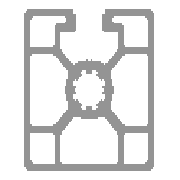
# Autodesk Inventor part: 3 842 992 401-25mm
Saved by Autodesk Inventor 2011 SP1 (Build 150282100, 282)
## iProperties
Category: End -/-
Created: 2011-02-21
Part Number: 3 842 992 401-25mm
Document SubType Name: Modeling
Designer: SRW
Density: 2.71 g/cm^3
Categories: <MemberInstance><Categories><Category DisplayName="Structural Shapes" InternalName="089c4875-fa83-4c05-b084-43b9cc11f5ed" Mnemonic="GRDR"><CategoryParameter DisplayName="Custom Base Point" InternalName="4f1d1b73-316d-484b-a3df-9cbabb16eb77" Mnemonic="shpBasePoint"/><CategoryParameter DisplayName="FG Authored" InternalName="9c666724-f362-4ea7-ac62-f6a007de5c69" Mnemonic="shpFGAuto"/><CategoryParameter DisplayName="Legacy Member ID" InternalName="340afe4f-75d7-48d3-ab7d-943f3c3da468" Mnemonic="LegacyMemberID"/><CategoryParameter DisplayName="Base Length" InternalName="42e34263-8f20-4d0e-ad48-bf1385b87c24" Mnemonic="shplen"/><CategoryParameter DisplayName="Distance of the Center of Gravity X-X" InternalName="26c9bdb8-9c79-4b4f-a92e-8e197583c9c4" Mnemonic="grcendistX"/><CategoryParameter DisplayName="Distance of the Center of Gravity Y-Y" InternalName="bcc4fb17-7af4-436a-8f8c-d0aa3b0248c5" Mnemonic="grcendistY"/><CategoryParameter DisplayName="Torsional Rigidity Modulus" InternalName="26c1ec35-5026-4c63-ad0a-751cf684a536" Mnemonic="torrigmod"/><CategoryParameter DisplayName="Torsional Section Modulus" InternalName="7c55a8dc-8844-49f9-a867-cc677b30ec9a" Mnemonic="torsecmod"/><CategoryParameter DisplayName="Coefficient of Shear Displacement" InternalName="de4c90c6-aaa8-468f-a335-6737b311b5d3" Mnemonic="shdispc"/><CategoryParameter DisplayName="Section Area" InternalName="1ff91680-64b0-4202-b9a3-7fd3f94bba3b" Mnemonic="secarea"/><CategoryParameter DisplayName="Moment of Inertia (x)" InternalName="4cd780bc-73d7-43ac-917a-579e5cbd684d" Mnemonic="inermomx"/><CategoryParameter DisplayName="Moment of Inertia (y)" InternalName="4b9f58ea-bced-460e-81ea-3d29ca5a49e3" Mnemonic="inermomy"/><CategoryParameter DisplayName="Section Module (x)" InternalName="72cfad18-cf51-4ed4-aaa7-c6b224f8419f" Mnemonic="secmodx"/><CategoryParameter DisplayName="Section Module (y)" InternalName="59eaa5e9-d227-48dc-b6c1-6920f96e0f95" Mnemonic="secmody"/><CategoryParameter DisplayName="Radius of Gyration (x)" InternalName="25778675-03e9-40c1-b6a8-4a9ed693320d" Mnemonic="gyrradx"/><CategoryParameter DisplayName="Radius of Gyration (y)" InternalName="bfa18ebe-1636-4dbe-8d42-b263e0b73184" Mnemonic="gyrrady"/><CategoryParameter DisplayName="Shape Thickness" InternalName="d109cf76-8eb4-42fc-9800-4409734adc67" Mnemonic="shpthick"/><CategoryParameter DisplayName="Second Shape Thickness" InternalName="9251a8e1-85fd-4e47-af99-afdb762317d9" Mnemonic="shpthick2"/><CategoryParameter DisplayName="Shape Width" InternalName="7c717d54-a18f-4666-b4d4-573cce22c62c" Mnemonic="shpwdth"/><CategoryParameter DisplayName="Shape Height" InternalName="50274e7d-5ac0-4796-92cb-c59e54983c67" Mnemonic="shpheig"/><CategoryParameter DisplayName="Mass per Length Unit" InternalName="0bb95a10-148f-4027-a459-38d7b056702a" Mnemonic="shpmass"/><CategoryParameter DisplayName="Section Designation" InternalName="5a64d034-428d-49c8-ba32-7619764de20f" Mnemonic="shpdes"/><Category DisplayName="Other" InternalName="f02205ff-2390-476f-921c-0b3185f88e84" Mnemonic="OTHSHP"><CategoryParameter DisplayName="Moment of Inertia (x)" InternalName="ec6737bc-264f-43ed-b0bd-f6d410c2718d" Mnemonic="inermomx"/><CategoryParameter DisplayName="Moment of Inertia (y)" InternalName="044c654e-f649-48ac-84cc-650a29ae31ca" Mnemonic="inermomy"/><CategoryParameter DisplayName="Section Module (x)" InternalName="cac70804-9d39-43bb-be17-56ea1f39a6c2" Mnemonic="secmodx"/><CategoryParameter DisplayName="Section Module (y)" InternalName="88b8bff9-a616-4028-93d5-ed4f79680d13" Mnemonic="secmody"/><CategoryParameter DisplayName="Section Area" InternalName="c46ecdf8-b6eb-4db9-8b25-30258930c1e3" Mnemonic="secarea"/><CategoryParameter DisplayName="Radius of Gyration (x)" InternalName="ee72c61e-565e-4fd6-b448-66e1e1abcb7e" Mnemonic="gyrradx"/><CategoryParameter DisplayName="Radius of Gyration (y)" InternalName="743e1dfe-1bba-408b-b985-cf752b207386" Mnemonic="gyrrady"/><CategoryParameter DisplayName="Shape Thickness" InternalName="12b1a788-9233-48fd-a933-2df8ff42b15f" Mnemonic="shpthick"/><CategoryParameter DisplayName="Mass per Length Unit" InternalName="2fd289d6-9394-4d2d-97e6-6659d7d4551d" Mnemonic="shpmass"/></Category></Category></Categories><FamilyTemplate Id="45x45 1S"><FamilyTemplateParameters><FamilyTemplateParameter ObjectType="kUserParameterObject" ValueType="xs:double" Id="9" ObjectReferenceKey="G_L"/><FamilyTemplateParameter ObjectType="kUserParameterObject" ValueType="xs:double" Id="10" ObjectReferenceKey="G_OFFSET_END"/><FamilyTemplateParameter ObjectType="kUserParameterObject" ValueType="xs:double" Id="11" ObjectReferenceKey="G_OFFSET_START"/><FamilyTemplateParameter ObjectType="kUserParameterObject" ValueType="xs:double" Id="12" ObjectReferenceKey="Length"/><FamilyTemplateParameter ObjectType="kPartFeatureObject" ValueType="xs:boolean" Id="1" ObjectReferenceKey="10020000100000001d0d0000000000008000000000000000" SubObjectId="Suppressed"/><FamilyTemplateParameter ObjectType="kPartFeatureObject" ValueType="xs:boolean" Id="2" ObjectReferenceKey="1002000010000000c00e0000000000008000000000000000" SubObjectId="Suppressed"/><FamilyTemplateParameter ObjectType="kPartFeatureObject" ValueType="xs:boolean" Id="3" ObjectReferenceKey="1002000010000000930f0000000000008000000000000000" SubObjectId="Suppressed"/><FamilyTemplateParameter ObjectType="kPartFeatureObject" ValueType="xs:boolean" Id="4" ObjectReferenceKey="1002000010000000180b0000000000008000000000000000" SubObjectId="Suppressed"/><FamilyTemplateParameter ObjectType="kPartFeatureObject" ValueType="xs:boolean" Id="6" ObjectReferenceKey="1002000010000000330c0000000000008000000000000000" SubObjectId="Suppressed"/><FamilyTemplateParameter ObjectType="kPartFeatureObject" ValueType="xs:boolean" Id="7" ObjectReferenceKey="1002000010000000f40d0000000000008000000000000000" SubObjectId="Suppressed"/><FamilyTemplateParameter ObjectType="kPartFeatureObject" ValueType="xs:boolean" Id="8" ObjectReferenceKey="10020000100000008b160000000000008000000000000000" SubObjectId="Suppressed"/><FamilyTemplateParameter ObjectType="kPartFeatureObject" ValueType="xs:boolean" Id="13" ObjectReferenceKey="1002000010000000590a0000000000008000000000000000" SubObjectId="Suppressed"/><FamilyTemplateParameter ObjectType="kPropertyObject" ValueType="xs:string" Id="16" ObjectReferenceKey="{D5CDD502-2E9C-101B-9397-08002B2CF9AE}" SubObjectId="2"/><FamilyTemplateParameter ObjectType="kPropertyObject" ValueType="xs:string" Id="17" ObjectReferenceKey="{32853F0F-3444-11d1-9E93-0060B03C1CA6}" SubObjectId="52"/><FamilyTemplateParameter ObjectType="kPartComponentDefinitionObject" ValueType="xs:string" Id="18" SubObjectId="Material"/><FamilyTemplateParameter ObjectType="kPropertyObject" ValueType="xs:string" Id="19" ObjectReferenceKey="{32853F0F-3444-11d1-9E93-0060B03C1CA6}" SubObjectId="5"/><FamilyTemplateParameter ObjectType="kPropertyObject" ValueType="xs:string" Id="20" ObjectReferenceKey="{32853F0F-3444-11D1-9E93-0060B03C1CA6}" SubObjectId="55"/><FamilyTemplateParameter ObjectType="kiPartTableColumnObject" ValueType="xs:string" Id="29" ObjectReferenceKey="FILENAME"/><FamilyTemplateParameter ObjectType="kiPartTableColumnObject" ValueType="xs:string" Id="30" ObjectReferenceKey="MEMBER_REVISION"/></FamilyTemplateParameters></FamilyTemplate><CategoryParameterMap><ParamToTemplateMap><ParamToTemplate CategoryParameter="//CategoryParameter[@InternalName='2675968c-4ce5-49e0-a4f5-552d29089031']" TemplateParameter="17"/><ParamToTemplate CategoryParameter="//CategoryParameter[@InternalName='8b46a4cc-9585-4fed-90c3-899f57e09a73']" TemplateParameter="29"/><ParamToTemplate CategoryParameter="//CategoryParameter[@InternalName='42e34263-8f20-4d0e-ad48-bf1385b87c24']" TemplateParameter="12"/><ParamToTemplate CategoryParameter="//CategoryParameter[@InternalName='818a152a-d3c3-49ca-80ee-df7d91421b8e']" TemplateParameter="18"/><ParamToTemplate CategoryParameter="//CategoryParameter[@InternalName='a65d44b9-392f-4f4f-857b-e4b3d54996fe']" TemplateParameter="30"/><ParamToTemplate CategoryParameter="//CategoryParameter[@InternalName='016b6077-bfbe-49bd-92c9-d8d59c39c941']" TemplateParameter="19"/><ParamToTemplate CategoryParameter="//CategoryParameter[@InternalName='9c666724-f362-4ea7-ac62-f6a007de5c69']" ConstantValue="1"/></ParamToTemplateMap></CategoryParameterMap></MemberInstance>
Stock Number: 3 842 992 401
Description: PROFILE 45x45 1S, -/-
Material: Aluminum-6061
Mass: 39.9838 g
Surface Area: 162.834 cm^2
Volume: 14.7542 cm^3
G_L: 25.000 mm
Author: SRW
Autodesk Inventor part; units mm, degrees
ref_plane "YZ Plane" through (0, 0, 0) normal (1, 0, 0) x (0, 1, 0)
ref_plane "XZ Plane" through (0, 0, 0) normal (0, 1, 0) x (-1, 0, 0)
sketch "45x45 1S" plane through (0, 0, 0) normal (0, 0, 1) x (1, 0, 0)
  line L0 (49.3347, 47.491) -> (36.1347, 47.491)
  arc A0 (36.1347, 47.491) -> (35.6347, 46.991) centre (36.1347, 46.991) ccw
  line L1 (35.6347, 46.991) -> (35.6347, 46.291)
  line L2 (35.3347, 45.991) -> (35.1347, 45.991)
  arc A1 (35.3347, 45.991) -> (35.6347, 46.291) centre (35.3347, 46.291) ccw
  line L3 (48.2375, 45.841) -> (38.8875, 45.841)
  arc A2 (35.1347, 45.991) -> (34.8347, 45.691) centre (35.1347, 45.691) ccw
  arc A3 (52.3347, 44.491) -> (49.3347, 47.491) centre (49.3347, 44.491) ccw
  arc A4 (50.7375, 43.341) -> (48.2375, 45.841) centre (48.2375, 43.341) ccw
  arc A5 (38.8875, 45.841) -> (38.8875, 43.141) centre (38.8875, 44.491) ccw
  line L4 (38.8875, 43.141) -> (40.5875, 43.141)
  line L5 (34.8347, 45.691) -> (34.8347, 41.691)
  arc A6 (34.8347, 41.691) -> (35.0347, 41.491) centre (35.0347, 41.691) ccw
  line L6 (35.0347, 41.491) -> (39.6847, 41.491)
  arc A7 (39.8847, 41.291) -> (39.6847, 41.491) centre (39.6847, 41.291) ccw
  line L7 (41.5875, 42.141) -> (41.5875, 37.691)
  line L8 (50.7375, 37.691) -> (50.7375, 43.341)
  line L9 (39.8847, 41.291) -> (39.8847, 36.8066)
  line L10 (42.5875, 36.691) -> (49.7375, 36.691)
  arc A8 (49.7375, 36.691) -> (50.7375, 37.691) centre (49.7375, 37.691) ccw
  arc A9 (41.5875, 37.691) -> (42.5875, 36.691) centre (42.5875, 37.691) ccw
  arc A10 (41.5875, 42.141) -> (40.5875, 43.141) centre (40.5875, 42.141) ccw
  line L11 (50.7375, 15.941) -> (50.7375, 34.041)
  arc A11 (50.7375, 34.041) -> (49.7375, 35.041) centre (49.7375, 34.041) ccw
  line L12 (49.7375, 35.041) -> (42.4984, 35.041)
  arc A12 (42.4984, 35.041) -> (41.0842, 34.4553) centre (42.4984, 33.041) ccw
  arc A13 (39.2989, 35.3924) -> (39.8847, 36.8066) centre (37.8847, 36.8066) ccw
  line L13 (41.0842, 34.4553) -> (37.447, 30.8181)
  arc A14 (37.447, 30.8181) -> (37.0665, 28.5213) centre (38.8612, 29.4039) ccw
  line L14 (39.2989, 35.3924) -> (36.4578, 32.5512)
  arc A15 (37.0665, 21.4608) -> (37.0665, 28.5213) centre (29.8875, 24.991) ccw
  line L15 (52.3347, 5.491) -> (52.3347, 44.491)
  arc A16 (30.7383, 32.991) -> (30.614, 32.9554) centre (30.7353, 32.767) ccw
  arc A17 (34.161, 32.1707) -> (30.7383, 32.991) centre (30.6307, 24.9918) ccw
  arc A18 (34.161, 32.1707) -> (36.4578, 32.5512) centre (35.0436, 33.9654) ccw
  arc A19 (35.7235, 23.3997) -> (35.3276, 24.0225) centre (35.2408, 23.5301) ccw
  arc A20 (35.3276, 25.9596) -> (35.7235, 26.5824) centre (35.2408, 26.452) ccw
  arc A21 (35.124, 21.9524) -> (35.7235, 23.3997) centre (29.8347, 24.991) ccw
  arc A22 (35.7235, 26.5824) -> (35.124, 28.0297) centre (29.8347, 24.991) ccw
  line L16 (34.81, 25.8683) -> (35.3276, 25.9596)
  line L17 (35.3276, 24.0225) -> (34.81, 24.1138)
  arc A23 (34.81, 24.1138) -> (34.81, 25.8683) centre (29.8875, 24.991) ccw
  arc A24 (34.4036, 21.7918) -> (35.124, 21.9524) centre (34.6904, 22.2014) ccw
  line L18 (34.4036, 28.1902) -> (33.9658, 27.8837)
  line L19 (33.9658, 22.0984) -> (34.4036, 21.7918)
  arc A25 (32.8734, 19.7018) -> (33.0339, 20.4221) centre (32.6243, 20.1353) ccw
  line L20 (33.0339, 20.4221) -> (32.7199, 20.8706)
  arc A26 (32.7199, 20.8706) -> (33.9658, 22.0984) centre (29.8875, 24.991) ccw
  arc A27 (31.4261, 19.1023) -> (32.8734, 19.7018) centre (29.8347, 24.991) ccw
  arc A28 (29.8347, 17.0144) -> (33.3735, 17.8163) centre (29.8875, 24.991) ccw
  arc A29 (30.8033, 19.4982) -> (31.4261, 19.1023) centre (31.2957, 19.585) ccw
  line L21 (30.703, 20.067) -> (30.8033, 19.4982)
  arc A30 (33.0867, 29.56) -> (32.8734, 30.2803) centre (32.6637, 29.8264) ccw
  arc A31 (33.9658, 27.8837) -> (32.7554, 29.0868) centre (29.8875, 24.991) ccw
  line L22 (32.7554, 29.0868) -> (33.0867, 29.56)
  arc A32 (32.8734, 30.2803) -> (31.4261, 30.8798) centre (29.8347, 24.991) ccw
  arc A33 (31.4261, 30.8798) -> (30.8033, 30.4839) centre (31.2957, 30.3971) ccw
  line L23 (30.8033, 30.4839) -> (30.7045, 29.9238)
  arc A34 (35.124, 28.0297) -> (34.4036, 28.1902) centre (34.6904, 27.7807) ccw
  arc A35 (49.3347, 2.491) -> (52.3347, 5.491) centre (49.3347, 5.491) ccw
  arc A36 (39.8847, 12.3802) -> (39.2989, 13.7944) centre (37.8847, 12.3802) ccw
  arc A37 (49.7375, 14.941) -> (50.7375, 15.941) centre (49.7375, 15.941) ccw
  line L24 (42.4984, 14.941) -> (49.7375, 14.941)
  arc A38 (41.0841, 15.5268) -> (42.4984, 14.941) centre (42.4984, 16.941) ccw
  line L25 (39.8847, 5.141) -> (39.8847, 12.3802)
  arc A39 (42.5875, 13.291) -> (41.5875, 12.291) centre (42.5875, 12.291) ccw
  line L26 (49.7375, 13.291) -> (42.5875, 13.291)
  arc A40 (50.7375, 12.291) -> (49.7375, 13.291) centre (49.7375, 12.291) ccw
  arc A41 (38.8847, 4.141) -> (39.8847, 5.141) centre (38.8847, 5.141) ccw
  line L27 (41.5875, 12.291) -> (41.5875, 5.141)
  arc A42 (41.5875, 5.141) -> (42.5875, 4.141) centre (42.5875, 5.141) ccw
  line L28 (50.7375, 6.641) -> (50.7375, 12.291)
  line L29 (42.5875, 4.141) -> (48.2375, 4.141)
  arc A43 (48.2375, 4.141) -> (50.7375, 6.641) centre (48.2375, 6.641) ccw
  arc A44 (23.2117, 32.5512) -> (25.5085, 32.1707) centre (24.6259, 33.9654) ccw
  arc A45 (28.9312, 32.991) -> (25.5085, 32.1707) centre (29.0387, 24.9918) ccw
  arc A46 (29.0555, 32.9554) -> (28.9312, 32.991) centre (28.9342, 32.767) ccw
  line L30 (29.7348, 32.5178) -> (29.0555, 32.9554)
  arc A47 (25.2658, 28.1902) -> (24.5455, 28.0297) centre (24.979, 27.7807) ccw
  arc A48 (26.796, 30.2803) -> (26.5827, 29.56) centre (27.0058, 29.8264) ccw
  line L31 (25.7036, 27.8837) -> (25.2658, 28.1902)
  arc A49 (29.7348, 32.5178) -> (29.8347, 32.491) centre (29.8348, 32.691) ccw
  arc A50 (29.8347, 32.491) -> (29.9347, 32.5178) centre (29.8347, 32.691) ccw
  line L32 (30.614, 32.9554) -> (29.9347, 32.5178)
  arc A51 (24.5455, 28.0297) -> (23.946, 26.5824) centre (29.8347, 24.991) ccw
  arc A52 (28.2433, 30.8798) -> (26.796, 30.2803) centre (29.8347, 24.991) ccw
  arc A53 (28.8662, 30.4839) -> (28.2433, 30.8798) centre (28.3738, 30.3971) ccw
  arc A54 (23.946, 26.5824) -> (24.3419, 25.9596) centre (24.4287, 26.452) ccw
  arc A55 (26.914, 29.0868) -> (25.7036, 27.8837) centre (29.7819, 24.991) ccw
  line L33 (28.965, 29.9238) -> (28.8662, 30.4839)
  line L34 (24.3419, 25.9596) -> (24.8595, 25.8683)
  arc A56 (29.8347, 29.9908) -> (28.965, 29.9238) centre (29.7819, 24.991) ccw
  arc A57 (30.7045, 29.9238) -> (29.8347, 29.9908) centre (29.8875, 24.991) ccw
  arc A58 (24.8595, 25.8683) -> (24.8595, 24.1138) centre (29.7819, 24.991) ccw
  line L35 (24.8595, 24.1138) -> (24.3419, 24.0225)
  arc A59 (24.3419, 24.0225) -> (23.946, 23.3997) centre (24.4287, 23.5301) ccw
  arc A60 (22.603, 28.5213) -> (22.603, 21.4608) centre (29.7819, 24.991) ccw
  arc A61 (23.946, 23.3997) -> (24.5455, 21.9524) centre (29.8347, 24.991) ccw
  arc A62 (24.5455, 21.9524) -> (25.2658, 21.7918) centre (24.979, 22.2014) ccw
  line L36 (25.2658, 21.7918) -> (25.7036, 22.0984)
  line L37 (26.5827, 29.56) -> (26.914, 29.0868)
  arc A63 (10.3347, 47.491) -> (7.3348, 44.491) centre (10.3347, 44.491) ccw
  line L38 (23.5348, 47.491) -> (10.3347, 47.491)
  arc A64 (24.0348, 46.991) -> (23.5348, 47.491) centre (23.5348, 46.991) ccw
  line L39 (24.0348, 46.291) -> (24.0348, 46.991)
  arc A65 (24.0348, 46.291) -> (24.3348, 45.991) centre (24.3348, 46.291) ccw
  line L40 (24.5348, 45.991) -> (24.3348, 45.991)
  arc A66 (24.8348, 45.691) -> (24.5348, 45.991) centre (24.5348, 45.691) ccw
  line L41 (24.8348, 41.691) -> (24.8348, 45.691)
  arc A67 (24.6348, 41.491) -> (24.8348, 41.691) centre (24.6348, 41.691) ccw
  line L42 (19.9848, 41.491) -> (24.6348, 41.491)
  arc A68 (19.9848, 41.491) -> (19.7848, 41.291) centre (19.9848, 41.291) ccw
  line L43 (19.7848, 36.8066) -> (19.7848, 41.291)
  arc A69 (19.7848, 36.8066) -> (20.3705, 35.3924) centre (21.7848, 36.8066) ccw
  arc A70 (17.0819, 36.691) -> (18.0819, 37.691) centre (17.0819, 37.691) ccw
  line L44 (18.0819, 37.691) -> (18.0819, 42.141)
  line L45 (9.9319, 36.691) -> (17.0819, 36.691)
  line L46 (19.0819, 43.141) -> (20.7819, 43.141)
  arc A71 (19.0819, 43.141) -> (18.0819, 42.141) centre (19.0819, 42.141) ccw
  arc A72 (8.9319, 37.691) -> (9.9319, 36.691) centre (9.9319, 37.691) ccw
  arc A73 (20.7819, 43.141) -> (20.7819, 45.841) centre (20.7819, 44.491) ccw
  line L47 (20.7819, 45.841) -> (11.4319, 45.841)
  arc A74 (11.4319, 45.841) -> (8.9319, 43.341) centre (11.4319, 43.341) ccw
  line L48 (8.9319, 43.341) -> (8.9319, 37.691)
  line L49 (10.3347, 2.491) -> (49.3347, 2.491)
  line L50 (37.447, 19.164) -> (41.0841, 15.5268)
  arc A75 (37.0665, 21.4608) -> (37.447, 19.164) centre (38.8612, 20.5782) ccw
  arc A76 (17.0819, 4.141) -> (18.0819, 5.141) centre (17.0819, 5.141) ccw
  arc A77 (18.0819, 12.291) -> (17.0819, 13.291) centre (17.0819, 12.291) ccw
  line L51 (18.0819, 5.141) -> (18.0819, 12.291)
  arc A78 (35.6618, 17.4316) -> (33.3735, 17.8163) centre (34.2476, 16.0174) ccw
  line L52 (39.2989, 13.7944) -> (35.6618, 17.4316)
  line L53 (20.7848, 4.141) -> (38.8847, 4.141)
  arc A79 (19.7848, 5.141) -> (20.7848, 4.141) centre (20.7848, 5.141) ccw
  line L54 (19.7848, 12.3802) -> (19.7848, 5.141)
  arc A80 (20.3705, 13.7944) -> (19.7848, 12.3802) centre (21.7848, 12.3802) ccw
  arc A81 (25.7036, 22.0984) -> (26.9496, 20.8706) centre (29.7819, 24.991) ccw
  arc A82 (28.9665, 20.067) -> (30.703, 20.067) centre (29.8347, 24.9911) ccw
  line L55 (26.9496, 20.8706) -> (26.6355, 20.4221)
  line L56 (28.8662, 19.4982) -> (28.9665, 20.067)
  arc A83 (26.796, 19.7018) -> (28.2433, 19.1023) centre (29.8347, 24.991) ccw
  arc A84 (28.2433, 19.1023) -> (28.8662, 19.4982) centre (28.3738, 19.585) ccw
  arc A85 (26.2959, 17.8163) -> (29.8347, 17.0144) centre (29.7819, 24.991) ccw
  arc A86 (22.2225, 19.164) -> (22.603, 21.4608) centre (20.8083, 20.5782) ccw
  arc A87 (26.2959, 17.8163) -> (24.0077, 17.4316) centre (25.4219, 16.0174) ccw
  line L57 (18.5853, 15.5268) -> (22.2225, 19.164)
  arc A88 (17.1711, 14.941) -> (18.5853, 15.5268) centre (17.1711, 16.941) ccw
  line L58 (24.0077, 17.4316) -> (20.3705, 13.7944)
  arc A89 (26.6355, 20.4221) -> (26.796, 19.7018) centre (27.0451, 20.1353) ccw
  arc A90 (7.3348, 5.491) -> (10.3347, 2.491) centre (10.3347, 5.491) ccw
  line L59 (7.3348, 44.491) -> (7.3348, 5.491)
  line L60 (23.2117, 32.5512) -> (20.3705, 35.3924)
  line L61 (11.4319, 4.141) -> (17.0819, 4.141)
  arc A91 (8.9319, 6.641) -> (11.4319, 4.141) centre (11.4319, 6.641) ccw
  line L62 (8.9319, 12.291) -> (8.9319, 6.641)
  arc A92 (9.9319, 13.291) -> (8.9319, 12.291) centre (9.9319, 12.291) ccw
  line L63 (17.0819, 13.291) -> (9.9319, 13.291)
  line L64 (9.9319, 14.941) -> (17.1711, 14.941)
  arc A93 (8.9319, 15.941) -> (9.9319, 14.941) centre (9.9319, 15.941) ccw
  line L65 (8.9319, 34.041) -> (8.9319, 15.941)
  line L66 (22.2225, 30.8181) -> (18.5853, 34.4553)
  arc A94 (18.5853, 34.4553) -> (17.1711, 35.041) centre (17.1711, 33.041) ccw
  line L67 (17.1711, 35.041) -> (9.9319, 35.041)
  arc A95 (9.9319, 35.041) -> (8.9319, 34.041) centre (9.9319, 34.041) ccw
  arc A96 (22.603, 28.5213) -> (22.2225, 30.8181) centre (20.8083, 29.4039) ccw
ref_plane "Start Plane" through (0, 0, 0) normal (0, 0, 1) x (1, 0, 0)
ref_plane "End Plane" through (0, 0, 25) normal (0, 0, 1) x (1, 0, 0)
sketch "Sketch1" plane through (0, 0, 0) normal (0, 0, 1) x (1, 0, 0)
  line L0 (19.5, 22.5) -> (6.3, 22.5)
  arc A0 (6.3, 22.5) -> (5.8, 22) centre (6.3, 22) ccw
  line L1 (5.8, 22) -> (5.8, 21.3)
  line L2 (5.5, 21) -> (5.3, 21)
  arc A1 (5.5, 21) -> (5.8, 21.3) centre (5.5, 21.3) ccw
  line L3 (18.4028, 20.85) -> (9.0528, 20.85)
  arc A2 (5.3, 21) -> (5, 20.7) centre (5.3, 20.7) ccw
  arc A3 (22.5, 19.5) -> (19.5, 22.5) centre (19.5, 19.5) ccw
  arc A4 (20.9028, 18.35) -> (18.4028, 20.85) centre (18.4028, 18.35) ccw
  arc A5 (9.0528, 20.85) -> (9.0528, 18.15) centre (9.0528, 19.5) ccw
  line L4 (9.0528, 18.15) -> (10.7528, 18.15)
  line L5 (5, 20.7) -> (5, 16.7)
  arc A6 (5, 16.7) -> (5.2, 16.5) centre (5.2, 16.7) ccw
  line L6 (5.2, 16.5) -> (9.85, 16.5)
  arc A7 (10.05, 16.3) -> (9.85, 16.5) centre (9.85, 16.3) ccw
  line L7 (11.7528, 17.15) -> (11.7528, 12.7)
  line L8 (20.9028, 12.7) -> (20.9028, 18.35)
  line L9 (10.05, 16.3) -> (10.05, 11.8156)
  line L10 (12.7528, 11.7) -> (19.9028, 11.7)
  arc A8 (19.9028, 11.7) -> (20.9028, 12.7) centre (19.9028, 12.7) ccw
  arc A9 (11.7528, 12.7) -> (12.7528, 11.7) centre (12.7528, 12.7) ccw
  arc A10 (11.7528, 17.15) -> (10.7528, 18.15) centre (10.7528, 17.15) ccw
  line L11 (20.9028, -9.05) -> (20.9028, 9.05)
  arc A11 (20.9028, 9.05) -> (19.9028, 10.05) centre (19.9028, 9.05) ccw
  line L12 (19.9028, 10.05) -> (12.6636, 10.05)
  arc A12 (12.6636, 10.05) -> (11.2494, 9.4642) centre (12.6636, 8.05) ccw
  arc A13 (9.4642, 10.4014) -> (10.05, 11.8156) centre (8.05, 11.8156) ccw
  line L13 (11.2494, 9.4642) -> (7.6123, 5.8271)
  arc A14 (7.6123, 5.8271) -> (7.2317, 3.5303) centre (9.0265, 4.4128) ccw
  line L14 (9.4642, 10.4014) -> (6.623, 7.5602)
  arc A15 (7.2317, -3.5303) -> (7.2317, 3.5303) centre (0.0528, 0) ccw
  line L15 (22.5, -19.5) -> (22.5, 19.5)
  arc A16 (0.9036, 8) -> (0.7792, 7.9643) centre (0.9006, 7.776) ccw
  arc A17 (4.3263, 7.1797) -> (0.9036, 8) centre (0.796, 0.0007) ccw
  arc A18 (4.3263, 7.1797) -> (6.623, 7.5602) centre (5.2088, 8.9744) ccw
  arc A19 (5.8887, -1.5914) -> (5.4929, -0.9685) centre (5.4061, -1.4609) ccw
  arc A20 (5.4929, 0.9685) -> (5.8887, 1.5914) centre (5.4061, 1.4609) ccw
  arc A21 (5.2892, -3.0387) -> (5.8887, -1.5914) centre (0, 0) ccw
  arc A22 (5.8887, 1.5914) -> (5.2892, 3.0387) centre (0, 0) ccw
  line L16 (4.9752, 0.8773) -> (5.4929, 0.9685)
  line L17 (5.4929, -0.9685) -> (4.9752, -0.8773)
  arc A23 (4.9752, -0.8773) -> (4.9752, 0.8773) centre (0.0528, 0) ccw
  arc A24 (4.5689, -3.1992) -> (5.2892, -3.0387) centre (4.8557, -2.7896) ccw
  line L18 (4.5689, 3.1992) -> (4.1311, 2.8926)
  line L19 (4.1311, -2.8926) -> (4.5689, -3.1992)
  arc A25 (3.0387, -5.2892) -> (3.1992, -4.5689) centre (2.7896, -4.8557) ccw
  line L20 (3.1992, -4.5689) -> (2.8851, -4.1204)
  arc A26 (2.8851, -4.1204) -> (4.1311, -2.8926) centre (0.0528, 0) ccw
  arc A27 (1.5914, -5.8887) -> (3.0387, -5.2892) centre (0, 0) ccw
  arc A28 (0, -7.9766) -> (3.5388, -7.1748) centre (0.0528, 0) ccw
  arc A29 (0.9685, -5.4929) -> (1.5914, -5.8887) centre (1.4609, -5.4061) ccw
  line L21 (0.8682, -4.924) -> (0.9685, -5.4929)
  arc A30 (3.252, 4.5689) -> (3.0387, 5.2892) centre (2.8289, 4.8354) ccw
  arc A31 (4.1311, 2.8926) -> (2.9207, 4.0958) centre (0.0528, 0) ccw
  line L22 (2.9207, 4.0958) -> (3.252, 4.5689)
  arc A32 (3.0387, 5.2892) -> (1.5914, 5.8887) centre (0, 0) ccw
  arc A33 (1.5914, 5.8887) -> (0.9685, 5.4929) centre (1.4609, 5.4061) ccw
  line L23 (0.9685, 5.4929) -> (0.8698, 4.9328)
  arc A34 (5.2892, 3.0387) -> (4.5689, 3.1992) centre (4.8557, 2.7896) ccw
  arc A35 (19.5, -22.5) -> (22.5, -19.5) centre (19.5, -19.5) ccw
  arc A36 (10.05, -12.6108) -> (9.4642, -11.1966) centre (8.05, -12.6108) ccw
  arc A37 (19.9028, -10.05) -> (20.9028, -9.05) centre (19.9028, -9.05) ccw
  line L24 (12.6636, -10.05) -> (19.9028, -10.05)
  arc A38 (11.2494, -9.4642) -> (12.6636, -10.05) centre (12.6636, -8.05) ccw
  line L25 (10.05, -19.85) -> (10.05, -12.6108)
  arc A39 (12.7528, -11.7) -> (11.7528, -12.7) centre (12.7528, -12.7) ccw
  line L26 (19.9028, -11.7) -> (12.7528, -11.7)
  arc A40 (20.9028, -12.7) -> (19.9028, -11.7) centre (19.9028, -12.7) ccw
  arc A41 (9.05, -20.85) -> (10.05, -19.85) centre (9.05, -19.85) ccw
  line L27 (11.7528, -12.7) -> (11.7528, -19.85)
  arc A42 (11.7528, -19.85) -> (12.7528, -20.85) centre (12.7528, -19.85) ccw
  line L28 (20.9028, -18.35) -> (20.9028, -12.7)
  line L29 (12.7528, -20.85) -> (18.4028, -20.85)
  arc A43 (18.4028, -20.85) -> (20.9028, -18.35) centre (18.4028, -18.35) ccw
  arc A44 (-6.623, 7.5602) -> (-4.3263, 7.1797) centre (-5.2088, 8.9744) ccw
  arc A45 (-0.9036, 8) -> (-4.3263, 7.1797) centre (-0.796, 0.0007) ccw
  arc A46 (-0.7792, 7.9643) -> (-0.9036, 8) centre (-0.9006, 7.776) ccw
  line L30 (-0.1, 7.5268) -> (-0.7792, 7.9643)
  arc A47 (-4.5689, 3.1992) -> (-5.2892, 3.0387) centre (-4.8557, 2.7896) ccw
  arc A48 (-3.0387, 5.2892) -> (-3.252, 4.5689) centre (-2.8289, 4.8354) ccw
  line L31 (-4.1311, 2.8926) -> (-4.5689, 3.1992)
  arc A49 (-0.1, 7.5268) -> (0, 7.5) centre (0, 7.7) ccw
  arc A50 (0, 7.5) -> (0.1, 7.5268) centre (0, 7.7) ccw
  line L32 (0.7792, 7.9643) -> (0.1, 7.5268)
  arc A51 (-5.2892, 3.0387) -> (-5.8887, 1.5914) centre (0, 0) ccw
  arc A52 (-1.5914, 5.8887) -> (-3.0387, 5.2892) centre (0, 0) ccw
  arc A53 (-0.9685, 5.4929) -> (-1.5914, 5.8887) centre (-1.4609, 5.4061) ccw
  arc A54 (-5.8887, 1.5914) -> (-5.4929, 0.9685) centre (-5.4061, 1.4609) ccw
  arc A55 (-2.9207, 4.0958) -> (-4.1311, 2.8926) centre (-0.0528, 0) ccw
  line L33 (-0.8698, 4.9328) -> (-0.9685, 5.4929)
  line L34 (-5.4929, 0.9685) -> (-4.9752, 0.8773)
  arc A56 (0, 4.9997) -> (-0.8698, 4.9328) centre (-0.0528, 0) ccw
  arc A57 (0.8698, 4.9328) -> (0, 4.9997) centre (0.0528, 0) ccw
  arc A58 (-4.9752, 0.8773) -> (-4.9752, -0.8773) centre (-0.0528, 0) ccw
  line L35 (-4.9752, -0.8773) -> (-5.4929, -0.9685)
  arc A59 (-5.4929, -0.9685) -> (-5.8887, -1.5914) centre (-5.4061, -1.4609) ccw
  arc A60 (-7.2317, 3.5303) -> (-7.2317, -3.5303) centre (-0.0528, 0) ccw
  arc A61 (-5.8887, -1.5914) -> (-5.2892, -3.0387) centre (0, 0) ccw
  arc A62 (-5.2892, -3.0387) -> (-4.5689, -3.1992) centre (-4.8557, -2.7896) ccw
  line L36 (-4.5689, -3.1992) -> (-4.1311, -2.8926)
  line L37 (-3.252, 4.5689) -> (-2.9207, 4.0958)
  arc A63 (-19.5, 22.5) -> (-22.5, 19.5) centre (-19.5, 19.5) ccw
  line L38 (-6.3, 22.5) -> (-19.5, 22.5)
  arc A64 (-5.8, 22) -> (-6.3, 22.5) centre (-6.3, 22) ccw
  line L39 (-5.8, 21.3) -> (-5.8, 22)
  arc A65 (-5.8, 21.3) -> (-5.5, 21) centre (-5.5, 21.3) ccw
  line L40 (-5.3, 21) -> (-5.5, 21)
  arc A66 (-5, 20.7) -> (-5.3, 21) centre (-5.3, 20.7) ccw
  line L41 (-5, 16.7) -> (-5, 20.7)
  arc A67 (-5.2, 16.5) -> (-5, 16.7) centre (-5.2, 16.7) ccw
  line L42 (-9.85, 16.5) -> (-5.2, 16.5)
  arc A68 (-9.85, 16.5) -> (-10.05, 16.3) centre (-9.85, 16.3) ccw
  line L43 (-10.05, 11.8156) -> (-10.05, 16.3)
  arc A69 (-10.05, 11.8156) -> (-9.4642, 10.4014) centre (-8.05, 11.8156) ccw
  arc A70 (-12.7528, 11.7) -> (-11.7528, 12.7) centre (-12.7528, 12.7) ccw
  line L44 (-11.7528, 12.7) -> (-11.7528, 17.15)
  line L45 (-19.9028, 11.7) -> (-12.7528, 11.7)
  line L46 (-10.7528, 18.15) -> (-9.0528, 18.15)
  arc A71 (-10.7528, 18.15) -> (-11.7528, 17.15) centre (-10.7528, 17.15) ccw
  arc A72 (-20.9028, 12.7) -> (-19.9028, 11.7) centre (-19.9028, 12.7) ccw
  arc A73 (-9.0528, 18.15) -> (-9.0528, 20.85) centre (-9.0528, 19.5) ccw
  line L47 (-9.0528, 20.85) -> (-18.4028, 20.85)
  arc A74 (-18.4028, 20.85) -> (-20.9028, 18.35) centre (-18.4028, 18.35) ccw
  line L48 (-20.9028, 18.35) -> (-20.9028, 12.7)
  line L49 (-19.5, -22.5) -> (19.5, -22.5)
  line L50 (7.6123, -5.827) -> (11.2494, -9.4642)
  arc A75 (7.2317, -3.5303) -> (7.6123, -5.827) centre (9.0265, -4.4128) ccw
  arc A76 (-12.7528, -20.85) -> (-11.7528, -19.85) centre (-12.7528, -19.85) ccw
  arc A77 (-11.7528, -12.7) -> (-12.7528, -11.7) centre (-12.7528, -12.7) ccw
  line L51 (-11.7528, -19.85) -> (-11.7528, -12.7)
  arc A78 (5.827, -7.5595) -> (3.5388, -7.1748) centre (4.4128, -8.9737) ccw
  line L52 (9.4642, -11.1966) -> (5.827, -7.5595)
  line L53 (-9.05, -20.85) -> (9.05, -20.85)
  arc A79 (-10.05, -19.85) -> (-9.05, -20.85) centre (-9.05, -19.85) ccw
  line L54 (-10.05, -12.6108) -> (-10.05, -19.85)
  arc A80 (-9.4642, -11.1966) -> (-10.05, -12.6108) centre (-8.05, -12.6108) ccw
  arc A81 (-4.1311, -2.8926) -> (-2.8851, -4.1204) centre (-0.0528, 0) ccw
  arc A82 (-0.8682, -4.924) -> (0.8682, -4.924) centre (0, 0) ccw
  line L55 (-2.8851, -4.1204) -> (-3.1992, -4.5689)
  line L56 (-0.9685, -5.4929) -> (-0.8682, -4.924)
  arc A83 (-3.0387, -5.2892) -> (-1.5914, -5.8887) centre (0, 0) ccw
  arc A84 (-1.5914, -5.8887) -> (-0.9685, -5.4929) centre (-1.4609, -5.4061) ccw
  arc A85 (-3.5388, -7.1748) -> (0, -7.9766) centre (-0.0528, 0) ccw
  arc A86 (-7.6123, -5.827) -> (-7.2317, -3.5303) centre (-9.0265, -4.4128) ccw
  arc A87 (-3.5388, -7.1748) -> (-5.827, -7.5595) centre (-4.4128, -8.9737) ccw
  line L57 (-11.2494, -9.4642) -> (-7.6123, -5.827)
  arc A88 (-12.6636, -10.05) -> (-11.2494, -9.4642) centre (-12.6636, -8.05) ccw
  line L58 (-5.827, -7.5595) -> (-9.4642, -11.1966)
  arc A89 (-3.1992, -4.5689) -> (-3.0387, -5.2892) centre (-2.7896, -4.8557) ccw
  arc A90 (-22.5, -19.5) -> (-19.5, -22.5) centre (-19.5, -19.5) ccw
  line L59 (-22.5, 19.5) -> (-22.5, -19.5)
  line L60 (-6.623, 7.5602) -> (-9.4642, 10.4014)
  line L61 (-18.4028, -20.85) -> (-12.7528, -20.85)
  arc A91 (-20.9028, -18.35) -> (-18.4028, -20.85) centre (-18.4028, -18.35) ccw
  line L62 (-20.9028, -12.7) -> (-20.9028, -18.35)
  arc A92 (-19.9028, -11.7) -> (-20.9028, -12.7) centre (-19.9028, -12.7) ccw
  line L63 (-12.7528, -11.7) -> (-19.9028, -11.7)
  line L64 (-19.9028, -10.05) -> (-12.6636, -10.05)
  arc A93 (-20.9028, -9.05) -> (-19.9028, -10.05) centre (-19.9028, -9.05) ccw
  line L65 (-20.9028, 9.05) -> (-20.9028, -9.05)
  line L66 (-7.6123, 5.8271) -> (-11.2494, 9.4642)
  arc A94 (-11.2494, 9.4642) -> (-12.6636, 10.05) centre (-12.6636, 8.05) ccw
  line L67 (-12.6636, 10.05) -> (-19.9028, 10.05)
  arc A95 (-19.9028, 10.05) -> (-20.9028, 9.05) centre (-19.9028, 9.05) ccw
  arc A96 (-7.2317, 3.5303) -> (-7.6123, 5.8271) centre (-9.0265, 4.4128) ccw
  constraints: 1 other
extrude "Body" add sketch "Sketch1" along normal up to surface (25 mm away) from surface at 0
sketch "Sketch47" plane through (0, 0, 0) normal (0, 0, 1) x (1, 0, 0)
  line L0 (0, 0) -> (10, 0)
ref_plane "Work Plane21" through (0, 0, 0) normal (0, -1, 0) x (1, 0, 0)
sketch "Sketch48" plane through (0, 0, 0) normal (0, -1, 0) x (1, 0, 0)
  line L0 (-31.5, 0) -> (31.5, 0)
  line L1 (-31.5, 25) -> (31.5, 25)
  dimension "d7" = 25
  measures "d7" distance between parallel lines of L0 L1
sketch "Sketch9" plane through (0, 0, 0) normal (0, 0, 1) x (1, 0, 0)
  point P0 (0, 0)
hole "M12/-" [suppressed]
sketch "Sketch10" plane through (0, 0, 25) normal (0, 0, 1) x (1, 0, 0)
  point P0 (0, 0)
hole "-/M12" [suppressed]
sketch "Sketch11" plane through (0, 0, 0) normal (0, 1, 0) x (-1, 0, 0)
  line L0 (-13.7, 0) -> (12.2, 0) projected
  circle A0 centre (0, 22.5) radius 8.5
  point P0 (0, 0)
  dimension "d31" = 22.5
  dimension "d32" = 17
  constraints: 1 centre point, 1 vertical alignment
  measures "d31" distance from line of A0.centre L0
  measures "d32" diameter of A0
extrude "D17/-" [suppressed]
sketch "Sketch12" plane through (0, 0, 0) normal (0, 1, 0) x (-1, 0, 0)
  line L0 (-13.7, 25) -> (12.2, 25) projected
  circle A0 centre (0, 2.5) radius 8.5
  point P0 (0, 0)
  dimension "d35" = 17
  dimension "d36" = 22.5
  constraints: 1 centre point, 1 vertical alignment
  measures "d35" diameter of A0
  measures "d36" distance from line of L0 A0.centre
extrude "-/D17" [suppressed]
sketch "Sketch13" plane through (0, 0, 0) normal (0, 1, 0) x (-1, 0, 0)
  line L0 (-12.98, 0) -> (7.88, 0) projected
  circle A0 centre (0, 22.5) radius 4.9
  point P0 (0, 0)
  dimension "d39" = 9.8
  dimension "d40" = 22.5
  constraints: 1 centre point, 1 vertical alignment
  measures "d39" diameter of A0
  measures "d40" distance from line of A0.centre L0
extrude "D9.8/-" [suppressed]
sketch "Sketch14" plane through (0, 0, 0) normal (0, 1, 0) x (-1, 0, 0)
  line L0 (-12.98, 25) -> (7.88, 25) projected
  circle A0 centre (0, 2.5) radius 4.9
  point P0 (0, 0)
  dimension "d43" = 9.8
  dimension "d44" = 22.5
  constraints: 1 centre point, 1 vertical alignment
  measures "d43" diameter of A0
  measures "d44" distance from line of L0 A0.centre
extrude "-/D9.8" [suppressed]
sketch "Sketch15" plane through (0, 0, 0) normal (1, 0, 0) x (0, 1, 0)
  line L0 (-6.86, 25) -> (6.86, 25) projected
  circle A0 centre (0, 2.5) radius 4.9
  point P0 (0, 0)
  dimension "d47" = 9.8
  dimension "d48" = 22.5
  constraints: 1 centre point, 1 vertical alignment
  measures "d47" diameter of A0
  measures "d48" distance from line of L0 A0.centre
extrude "-/D9.8VS" [suppressed]
sketch "Sketch26" plane through (0, 0, 0) normal (1, 0, 0) x (0, 1, 0)
  circle A0 centre (0, 22.5) radius 4.9
  line L0 (-6.86, 0) -> (6.86, 0) projected
  point P0 (0, 0)
  dimension "d62" = 9.8
  dimension "d65" = 22.5
  constraints: 1 centre point, 1 vertical alignment
  measures "d62" diameter of A0
  measures "d65" distance from line of L0 A0.centre
extrude "D9.8VS/-" [suppressed]
equation "\"G_OFFSET_START\" = 0"
equation "\"G_OFFSET_END\" = 0"
equation "\"d3\" = Length + G_OFFSET_END"
equation "\"G_L\" = d7"
equation "\"Length2\" = G_OFFSET_START + Length + G_OFFSET_END"
equation "\"Length\" = 25"
body "Solid1"
